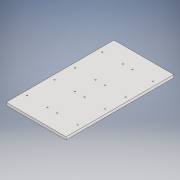
# Autodesk Inventor part: Fastener
Saved by Autodesk Inventor 2019.2 (Build 232265000, 265)
## iProperties
Created: 2020-05-06
Part Number: Fastener
Material: PC/ABS Plastic
Document SubType Name: Modeling
Designer: Johansson
Density: 0.357273 g/cm^3
Appearance: Smooth - White
Author: Johansson
Autodesk Inventor part; units mm, degrees
ref_plane "YZ Plane" through (0, 0, 0) normal (1, 0, 0) x (0, 1, 0)
ref_plane "XZ Plane" through (0, 0, 0) normal (0, 1, 0) x (-1, 0, 0)
ref_plane "XY Plane" through (0, 0, 0) normal (0, 0, 1) x (1, 0, 0)
sketch "Sketch1" plane through (0, 0, 0) normal (0, 1, 0) x (-1, 0, 0)
  line L0 (-87.5, 157.5) -> (87.5, 157.5)
  line L1 (87.5, 157.5) -> (87.5, -157.5)
  line L2 (87.5, -157.5) -> (-87.5, -157.5)
  line L3 (-87.5, -157.5) -> (-87.5, 157.5)
  line L4 (-87.5, 157.5) -> (87.5, -157.5) construction
  line L5 (87.5, 157.5) -> (-87.5, -157.5) construction
  point P0 (0, 0)
  dimension "d0" = 315
  dimension "d1" = 175
  constraints: 12 end point, 2 midpoint, 2 parallel, 1 horizontal, 1 perpendicular
  measures "d0" distance of L0.end L1.end
  measures "d1" distance between parallel lines of L3 L1
extrude "Extrusion1" add sketch "Sketch1" along normal blind 8
sketch "Sketch2" plane through (0, 8, 0) normal (0, 1, 0) x (1, 0, 0)
  circle A0 centre (-74, -110) radius 1.5
  line L0 (-87.5, 157.5) -> (-87.5, -157.5) projected
  line L1 (-87.5, -157.5) -> (87.5, -157.5) projected
  circle A1 centre (-74, -30) radius 1.5
  circle A2 centre (-14, -110) radius 1.5
  circle A3 centre (-14, -30) radius 1.5
  line L2 (-122.5, 0) -> (122.5, 0) projected
  line L3 (0, 220.5) -> (0, -220.5) projected
  circle A4 centre (-74, 110) radius 1.5
  circle A5 centre (-74, 30) radius 1.5
  circle A6 centre (-14, 110) radius 1.5
  circle A7 centre (-14, 30) radius 1.5
  circle A8 centre (74, -110) radius 1.5
  circle A9 centre (74, -30) radius 1.5
  circle A10 centre (14, -110) radius 1.5
  circle A11 centre (14, -30) radius 1.5
  circle A12 centre (74, 110) radius 1.5
  circle A13 centre (74, 30) radius 1.5
  circle A14 centre (14, 110) radius 1.5
  circle A15 centre (14, 30) radius 1.5
  point P0 (0, 0)
  dimension "d6" = 80
  dimension "d9" = 60
  dimension "d12" = 14
  dimension "d13" = 30
  dimension "d14" = 3
  constraints: 16 centre point, 12 symmetric about line, 1 horizontal, 1 vertical, 18 other
  measures "d6" distance of A0.centre A1.centre
  measures "d9" distance of A0.centre A2.centre
  measures "d12" distance from line of L3 A3.centre
  measures "d13" distance from line of L2 A3.centre
  measures "d14" diameter of A0
extrude "Extrusion2" cut sketch "Sketch2" against normal up to next contours A0 | A1 | A2 | A3 | A4 | A5 | A6 | A7 | A8 | A9 | A10 | A11 | A12 | A13 | A14 | A15
equation "\"d0\" = 3.5 * L_pcb_outer"
equation "\"d1\" = 2.5 * W_pcb_outer"
equation "\"d2\" = T_fastener"
equation "\"d6\" = L_pcb_holetohole"
equation "\"d9\" = W_pcb_holetohole"
equation "\"d12\" = 0.2 * W_pcb_outer"
equation "\"d13\" = 0.333333 * L_pcb_outer"
equation "\"d15\" = T_fastener"
equation "\"L_pcb_holetohole\" = 80"
equation "\"W_pcb_holetohole\" = 60"
equation "\"T_fastener\" = 8"
equation "\"L_pcb_outer\" = 90"
equation "\"W_pcb_outer\" = 70"
body "Solid1"
